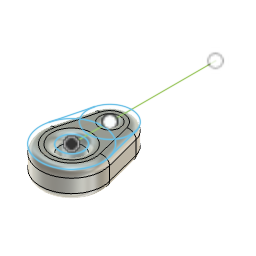
mmono (Autodesk Fusion 360 design; units mm, degrees)
Autodesk Fusion 360 part; units mm, degrees
sketch "Sketch1" plane through (0, 0, 0) normal (0, 0, 1) x (1, 0, 0)
  line L0 (0, -0.3827) -> (0, 150)
  circle A0 centre (0, -0.3827) radius 12.5
  circle A1 centre (0, -0.3827) radius 32.5
  circle A2 centre (0, 39.6173) radius 2.5
  circle A3 centre (0, 39.6173) radius 22.5
  line L1 (21.7855, 45.2423) -> (31.468, 7.7423)
  line L2 (-21.7855, 45.2423) -> (-31.468, 7.7423)
  dimension "d38" = 20
  dimension "d39" = 25
  dimension "d40" = 5
  dimension "d42" = 40
  dimension "d43" = 20
  constraint coincident L0.start A0.centre
  constraint coincident A3 L1.start
  constraint tangent A3 L1
  constraint coincident A1 L1.end
  constraint tangent A1 L1
  constraint coincident A3 L2.start
  constraint tangent A3 L2
  constraint coincident A1 L2.end
  constraint tangent A1 L2
  measures "d39" diameter of A0
  measures "d40" diameter of A2
  measures "d42" distance of L0.start A2.centre
extrude "Extrude6" add sketch "Sketch1" against normal blind 30 contours L0 A1 A3 | A1 A3 | L0 A1 A3 | L0 A1 A2 A3 | L0 A1 A2 A3 | A1 A3 L2 | A1 A3 L1 | A0
extrude "Extrude7" cut sketch "Sketch1" against normal blind 22.3431 contours A0
fillet "Fillet2" radius 8 11 edges at (-2.3308, 40.5214, 0) (0, -32.8827, 0) (-26.6268, 26.4923, 0) (0, 62.1173, 0) (26.6268, 26.4923, 0) (-11.6541, 4.1375, 0) (-2.3308, 38.7133, -30) (-26.6268, 26.4923, -30) (0, 62.1173, -30) (26.6268, 26.4923, -30) (0, -32.8827, -30)
